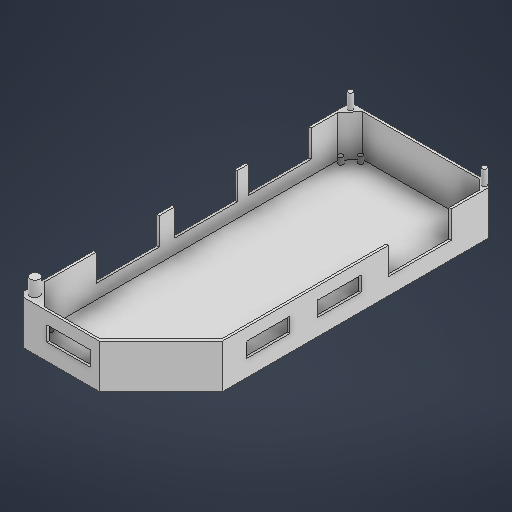
# Autodesk Inventor part: Bottom
Saved by Autodesk Inventor 2026.1 (Build 301233020, 233B)
## iProperties
Created: 2026-05-28
Part Number: Bottom
Material: Generic
Document SubType Name: Modeling
Designer: jcla0
Density: 1 g/cm^3
Appearance: Default
Author: jcla0
Autodesk Inventor part; units mm, degrees
ref_plane "YZ Plane" through (0, 0, 0) normal (1, 0, 0) x (0, 1, 0)
ref_plane "XZ Plane" through (0, 0, 0) normal (0, 1, 0) x (-1, 0, 0)
ref_plane "XY Plane" through (0, 0, 0) normal (0, 0, 1) x (1, 0, 0)
sketch "Sketch1" plane through (0, 0, 0) normal (0, 1, 0) x (-1, 0, 0)
  line L0 (21.5102, 17.7267) -> (21.5102, -43.9733)
  line L1 (21.5102, -43.9733) -> (19.1102, -46.7733)
  line L2 (19.1102, -46.7733) -> (-5.4898, -46.7733)
  line L3 (-5.4898, -46.7733) -> (-7.4898, -44.7733)
  line L4 (-7.4898, -44.7733) -> (-7.4898, 9.2267)
  line L5 (-7.4898, 9.2267) -> (5.5102, 22.2267)
  line L6 (5.5102, 22.2267) -> (17.0102, 22.2267)
  line L7 (17.0102, 22.2267) -> (21.5102, 17.7267)
  line L8 (22.0102, 21.7267) -> (22.0102, -46.2733)
  line L9 (22.0102, -46.2733) -> (21.0102, -47.2733)
  line L10 (21.0102, -47.2733) -> (-6.9898, -47.2733)
  line L11 (-6.9898, -47.2733) -> (-7.9898, -46.2733)
  line L12 (-7.9898, -46.2733) -> (-7.9898, 9.7267)
  line L13 (-7.9898, 9.7267) -> (5.0102, 22.7267)
  line L14 (5.0102, 22.7267) -> (21.0102, 22.7267)
  line L15 (21.0102, 22.7267) -> (22.0102, 21.7267)
  point P0 (0, 0)
  point P1 (14.1019, -14.4492)
  dimension "d0" = 69
  dimension "d1" = 29
  dimension "d2" = 2
  dimension "d3" = 2
  dimension "d4" = 2.8
  dimension "d5" = 2.4
  dimension "d6" = 4.5
  dimension "d7" = 4.5
  dimension "d8" = 13
  dimension "d9" = 13
  dimension "d10" = 70
  dimension "d11" = 30
  dimension "d12" = 1
  dimension "d13" = 1
  dimension "d14" = 1
  dimension "d15" = 1
  dimension "d16" = 1
  dimension "d17" = 1
  dimension "d18" = 13
  dimension "d19" = 13
  dimension "d34" = 0.5
  dimension "d35" = 0.5
  constraints: 32 end point, 4 parallel, 2 perpendicular, 2 vertical
  measures "d0" distance between parallel lines of L2 L6
  measures "d1" distance between parallel lines of L0 L4
  measures "d2" horizontal distance of L2.end L3.end
  measures "d3" horizontal distance of L2.end L3.end
  measures "d4" vertical distance of L1.end L0.end
  measures "d5" horizontal distance of L1.end L0.end
  measures "d6" horizontal distance of L0.start L6.end
  measures "d7" horizontal distance of L0.start L6.end
  measures "d8" horizontal distance of L4.end L5.end
  measures "d9" horizontal distance of L4.end L5.end
  measures "d10" distance between parallel lines of L10 L14
  measures "d11" distance between parallel lines of L8 L12
  measures "d12" horizontal distance of L10.end L11.end
  measures "d13" horizontal distance of L10.end L11.end
  measures "d14" horizontal distance of L9.end L8.end
  measures "d15" horizontal distance of L9.end L8.end
  measures "d16" horizontal distance of L8.start L14.end
  measures "d17" horizontal distance of L8.start L14.end
  measures "d18" horizontal distance of L12.end L13.end
  measures "d19" horizontal distance of L12.end L13.end
  measures "d34" distance between parallel lines of L14 L6
  measures "d35" distance between parallel lines of L12 L4
extrude "Extrusion1" add sketch "Sketch1" along normal blind 0.5 contours L0 L1 L2 L3 L4 L5 L6 L7 | L8 L9 L10 L11 L12 L13 L14 L15
extrude "Extrusion2" add sketch "Sketch1" along normal blind 9.2
sketch "Sketch2" plane through (0, 0.5, 0) normal (0, 1, 0) x (1, 0, 0)
  circle A0 centre (-20.6484, -17.3121) radius 0.5
  circle A1 centre (-16.6313, -21.3691) radius 0.5
  circle A2 centre (-5.7074, -21.3691) radius 0.5
  circle A3 centre (6.7103, -8.921) radius 0.5
  circle A4 centre (6.7103, 44.2469) radius 0.5
  circle A5 centre (5.3281, 46.0012) radius 0.5
  circle A6 centre (-20.6484, 43.7469) radius 0.5
  circle A7 centre (-18.7007, 46.0012) radius 0.5
  point P0 (0, 0)
  dimension "d24" = 1
  dimension "d25" = 1
  dimension "d26" = 1
  dimension "d27" = 1
  dimension "d28" = 1
  dimension "d29" = 1
  dimension "d30" = 1
  dimension "d31" = 1
  constraints: 8 centre point
  measures "d24" diameter of A0
  measures "d25" diameter of A1
  measures "d26" diameter of A2
  measures "d27" diameter of A3
  measures "d28" diameter of A4
  measures "d29" diameter of A5
  measures "d30" diameter of A6
  measures "d31" diameter of A7
extrude "Extrusion3" add sketch "Sketch2" along normal blind 1.4
sketch "Sketch3" plane through (0, 9.2, 0) normal (0, 1, 0) x (1, 0, 0)
  line L0 (-21.0102, -22.7267) -> (-5.0102, -22.7267) projected
  line L1 (-5.0102, -22.7267) -> (7.9898, -9.7267) projected
  line L2 (7.9898, -9.7267) -> (7.9898, 46.2733) projected
  line L3 (7.9898, 46.2733) -> (6.9898, 47.2733) projected
  line L4 (6.9898, 47.2733) -> (-21.0102, 47.2733) projected
  line L5 (-21.0102, 47.2733) -> (-22.0102, 46.2733) projected
  line L6 (-22.0102, 46.2733) -> (-22.0102, -21.7267) projected
  line L7 (-22.0102, -21.7267) -> (-21.0102, -22.7267) projected
  line L8 (-21.5102, -17.7267) -> (-21.5102, 43.9733) projected
  line L9 (-19.1102, 46.7733) -> (5.4898, 46.7733) projected
  line L10 (7.4898, 44.7733) -> (7.4898, -9.2267) projected
  line L11 (7.4898, -9.2267) -> (-5.5102, -22.2267) projected
  line L12 (-5.5102, -22.2267) -> (-17.0102, -22.2267) projected
  line L13 (-17.0102, -22.2267) -> (-21.5102, -17.7267) projected
  line L14 (-5.5102, -22.2267) -> (-17.0102, -22.2267) projected
  line L15 (-21.0102, -22.7267) -> (-5.0102, -22.7267) projected
  line L16 (-16.0102, -22.2267) -> (-6.9102, -22.2267)
  line L17 (-6.9102, -22.2267) -> (-6.9102, -22.7267)
  line L18 (-6.9102, -22.7267) -> (-16.0102, -22.7267)
  line L19 (-16.0102, -22.7267) -> (-16.0102, -22.2267)
  line L20 (-21.5102, 43.9733) -> (-19.1102, 46.7733) projected
  line L21 (5.4898, 46.7733) -> (7.4898, 44.7733) projected
  line L22 (7.4898, -4.7267) -> (7.9898, -4.7267)
  line L23 (7.9898, -4.7267) -> (7.9898, 4.3733)
  line L24 (7.9898, 4.3733) -> (7.4898, 4.3733)
  line L25 (7.4898, 4.3733) -> (7.4898, -4.7267)
  line L26 (7.4898, 10.2733) -> (7.9898, 10.2733)
  line L27 (7.9898, 10.2733) -> (7.9898, 19.3733)
  line L28 (7.9898, 19.3733) -> (7.4898, 19.3733)
  line L29 (7.4898, 19.3733) -> (7.4898, 10.2733)
  line L30 (7.4898, 25.1733) -> (7.9898, 25.1733)
  line L31 (7.9898, 25.1733) -> (7.9898, 38.3733)
  line L32 (7.9898, 38.3733) -> (7.4898, 38.3733)
  line L33 (7.4898, 38.3733) -> (7.4898, 25.1733)
  line L34 (-22.0102, -6.8267) -> (-21.5102, -6.8267)
  line L35 (-21.5102, -6.8267) -> (-21.5102, 6.3733)
  line L36 (-21.5102, 6.3733) -> (-22.0102, 6.3733)
  line L37 (-22.0102, 6.3733) -> (-22.0102, -6.8267)
  line L38 (-21.5102, 43.9733) -> (-21.5102, -17.7267) projected
  line L39 (-22.0102, 9.6733) -> (-21.5102, 9.6733)
  line L40 (-21.5102, 9.6733) -> (-21.5102, 22.8733)
  line L41 (-21.5102, 22.8733) -> (-22.0102, 22.8733)
  line L42 (-22.0102, 22.8733) -> (-22.0102, 9.6733)
  line L43 (-22.0102, 25.1733) -> (-21.5102, 25.1733)
  line L44 (-21.5102, 25.1733) -> (-21.5102, 38.3733)
  line L45 (-21.5102, 38.3733) -> (-22.0102, 38.3733)
  line L46 (-22.0102, 38.3733) -> (-22.0102, 25.1733)
  point P0 (0, 0)
  point P1 (-16.0102, -22.4767)
  point P2 (-6.9102, -22.4767)
  point P3 (7.7398, -4.7267)
  point P4 (7.7398, 4.3733)
  point P5 (7.7398, 19.3733)
  point P6 (7.7398, 10.2733)
  point P7 (7.7398, 25.1733)
  point P8 (7.7398, 38.3733)
  point P9 (-21.7602, 6.3733)
  point P10 (-21.7602, -6.8267)
  point P11 (-21.7602, 9.6733)
  point P12 (-21.7602, 22.8733)
  point P13 (-21.7602, 38.3733)
  point P14 (-21.7602, 25.1733)
  dimension "d36" = 1
  dimension "d37" = 1.4
  dimension "d38" = 4.5
  dimension "d39" = 9.1
  dimension "d40" = 5.7462
  dimension "d41" = 5.9
  dimension "d42" = 9.1
  dimension "d43" = 5.8
  dimension "d44" = 13.2
  dimension "d45" = 13.2
  dimension "d46" = 10.9
  dimension "d47" = 3.3
  dimension "d48" = 13.2
  dimension "d49" = 13.2
  dimension "d50" = 2.3
  constraints: 56 end point, 14 midpoint, 14 parallel, 14 point on line, 7 horizontal, 7 perpendicular
  measures "d36" horizontal distance of point (-16.01, -22.477) L12.end
  measures "d37" horizontal distance of L11.end point (-6.91, -22.477)
  measures "d38" distance from line of L10.end L22
  measures "d39" distance of point (7.74, -4.727) point (7.74, 4.373)
  measures "d41" distance from line of point (7.74, 4.373) L26
  measures "d42" distance of point (7.74, 19.373) point (7.74, 10.273)
  measures "d43" distance of point (7.74, 25.173) point (7.74, 19.373)
  measures "d44" distance of point (7.74, 25.173) point (7.74, 38.373)
  measures "d45" distance of point (-21.76, 6.373) point (-21.76, -6.827)
  measures "d46" vertical distance of L8.start point (-21.76, -6.827)
  measures "d47" distance of point (-21.76, 9.673) point (-21.76, 6.373)
  measures "d48" distance of point (-21.76, 9.673) point (-21.76, 22.873)
  measures "d49" distance of point (-21.76, 38.373) point (-21.76, 25.173)
  measures "d50" distance of point (-21.76, 25.173) point (-21.76, 22.873)
extrude "Extrusion4" cut sketch "Sketch3" against normal blind 5.7 contours L19 L12 L17 L0 | L6 L36 L8 L34 | L6 L41 L8 L39 | L22 L10 L24 L2 | L6 L45 L8 L43 | L26 L10 L28 L2 | L30 L10 L32 L2
sketch "Sketch4" plane through (0, 9.2, 0) normal (0, 1, 0) x (1, 0, 0)
  line L0 (-6.9102, -22.7267) -> (-16.0102, -22.7267) projected
  line L1 (-6.9102, -22.2267) -> (-6.9102, -22.7267) projected
  line L2 (-16.0102, -22.2267) -> (-6.9102, -22.2267) projected
  line L3 (-16.0102, -22.7267) -> (-16.0102, -22.2267) projected
  line L4 (7.4898, -4.7267) -> (7.4898, 4.3733) projected
  line L5 (7.9898, -4.7267) -> (7.4898, -4.7267) projected
  line L6 (7.9898, 4.3733) -> (7.9898, -4.7267) projected
  line L7 (7.4898, 4.3733) -> (7.9898, 4.3733) projected
  line L8 (7.4898, 10.2733) -> (7.4898, 19.3733) projected
  line L9 (7.9898, 10.2733) -> (7.4898, 10.2733) projected
  line L10 (7.9898, 19.3733) -> (7.9898, 10.2733) projected
  line L11 (7.4898, 19.3733) -> (7.9898, 19.3733) projected
  point P0 (0, 0)
extrude "Extrusion5" add sketch "Sketch4" against normal blind 2.54
sketch "Sketch5" plane through (0, 9.2, 0) normal (0, 1, 0) x (1, 0, 0)
  circle A0 centre (-20.3864, -20.9025) radius 1
  circle A1 centre (-20.8742, 46.0372) radius 0.5
  circle A2 centre (7.0371, 46.2575) radius 0.5
  point P0 (0, 0)
  dimension "d55" = 2
  dimension "d56" = 1
  dimension "d57" = 1
  constraints: 3 centre point
  measures "d55" diameter of A0
  measures "d56" diameter of A1
  measures "d57" diameter of A2
extrude "Extrusion6" add sketch "Sketch5" along normal blind 3.175
equation "\"d9\" = d8"
equation "\"d19\" = d18"
body "Solid1"
